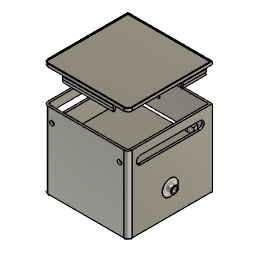
Chassis - Blank (Autodesk Fusion 360 design; units mm, degrees)
Autodesk Fusion 360 part; units mm, degrees
sketch "Floors" plane through (0, 0, 0) normal (0, 1, 0) x (1, 0, 0)
  line L0 (125, 0) -> (175, 0)
  line L1 (125, 2.5) -> (150, 2.5) construction
  line L2 (125, -23) -> (175, -23)
  line L3 (125, -20.5) -> (150, -20.5) construction
  line L4 (125, -22) -> (150, -22) construction
  line L5 (125, -35.125) -> (175, -35.125)
  line L6 (125, -36.725) -> (150, -36.725) construction
  line L7 (125, -36.125) -> (150, -36.125) construction
  line L8 (125, -55) -> (175, -55)
  line L9 (125, -52.5) -> (150, -52.5) construction
  line L10 (125, -62.5) -> (150, -62.5) construction
  line L11 (125, -90) -> (175, -90)
  line L12 (120, -130) -> (180, -130) construction
  line L13 (150, -4) -> (125, -4) construction
  line L14 (150, 1) -> (125, 1) construction
  line L15 (125, 3.5) -> (150, 3.5)
  dimension "d1" = 2.5
  dimension "d9" = 23
  dimension "d10" = 2.5
  dimension "d11" = 1
  dimension "d12" = 12.125
  dimension "d13" = 1
  dimension "d14" = 1.6
  dimension "d15" = 55
  dimension "d16" = 2.5
  dimension "d17" = 7.5
  dimension "d18" = 90
  dimension "d28" = 4
  dimension "d29" = 1
  dimension "d170" = 1
  constraint horizontal L0
  constraint horizontal L1
  constraint horizontal L2
  constraint parallel L2 L3
  constraint parallel L3 L4
  constraint horizontal L5
  constraint horizontal L6
  constraint horizontal L7
  constraint horizontal L8
  constraint horizontal L9
  constraint horizontal L10
  constraint horizontal L11
  constraint parallel L11 L12
  constraint parallel L5 L13
  constraint parallel L1 L14
  constraint horizontal L15
  measures "d1" distance of L0 L1
  measures "d9" distance of L0 L2
  measures "d10" distance of L2 L3
  measures "d11" distance of L2 L4
  measures "d12" distance of L2 L5
  measures "d13" distance of L5 L7
  measures "d14" distance of L5 L6
  measures "d15" distance of L0 L8
  measures "d16" distance of L8 L9
  measures "d17" distance of L8 L10
  measures "d18" distance of L0 L11
  measures "d28" distance of L0 L13
  measures "d29" distance of L0 L14
  measures "d170" distance of L1 L15
sketch "Base" plane through (0, 0, 0) normal (0, 0, 1) x (1, 0, 0)
  line L0 (-50, 50) -> (50, 50)
  line L1 (50, 50) -> (50, -50)
  line L2 (50, -50) -> (-50, -50)
  line L3 (-50, -50) -> (-50, 50)
  line L4 (-50, 50) -> (50, -50) construction
  line L5 (50, 50) -> (-50, -50) construction
  line L6 (47.5, -47.5) -> (-47.5, -47.5)
  line L7 (-47.5, -47.5) -> (-47.5, 47.5)
  line L8 (-47.5, 47.5) -> (47.5, 47.5)
  line L9 (47.5, 47.5) -> (47.5, -47.5)
  line L10 (47.5, -47.5) -> (-47.5, 47.5) construction
  line L11 (-47.5, -47.5) -> (47.5, 47.5) construction
  dimension "d4" = 100
  dimension "d6" = 95
  constraint horizontal L0
  constraint perpendicular L0 L1
  constraint parallel L0 L2
  constraint parallel L1 L3
  constraint coincident L4 origin
  constraint coincident L5 origin
  constraint horizontal L6
  constraint perpendicular L6 L7
  constraint parallel L6 L8
  constraint parallel L7 L9
  constraint coincident L10 origin
  constraint coincident L11 origin
  constraint coincident L4 L6.start
  constraint equal L0 L3
  measures "d4" distance of L0.start L0.end
  measures "d6" distance of L7.end L8.end
extrude "Extrude1" add sketch "Base" against normal up to surface (2.5 mm away) contours L0 L1 L2 L3 | L6 L7 L8 L9 makes body 1
extrude "Extrude2" add sketch "Base" along normal up to surface (90 mm away) bodies 1
fillet "Fillet1" radius 5 2 edges at (-50, -50, 43.75) (50, -50, 43.75) on bodies 1
sketch "Battery Mount" plane through (0, 0, 0) normal (0, 0, 1) x (1, 0, 0)
  line L0 (-15.5, 30) -> (15.5, 30)
  line L1 (15.5, 30) -> (15.5, -30)
  line L2 (15.5, -30) -> (-15.5, -30)
  line L3 (-15.5, -30) -> (-15.5, 30)
  line L4 (-15.5, 30) -> (15.5, -30) construction
  line L5 (15.5, 30) -> (-15.5, -30) construction
  line L6 (17.5, 32) -> (-17.5, 32)
  line L7 (-17.5, 32) -> (-17.5, -32)
  line L8 (-17.5, -32) -> (17.5, -32)
  line L9 (17.5, -32) -> (17.5, 32)
  line L10 (17.5, 32) -> (-17.5, -32) construction
  line L11 (-17.5, 32) -> (17.5, -32) construction
  line L12 (15.5, 30) -> (15.5, 32)
  line L13 (-15.5, 30) -> (-15.5, 32)
  dimension "d23" = 31
  dimension "d24" = 60
  dimension "d26" = 2
  dimension "d27" = 2
  constraint horizontal L0
  constraint perpendicular L0 L1
  constraint parallel L0 L2
  constraint parallel L1 L3
  constraint coincident L4 origin
  constraint coincident L5 origin
  constraint horizontal L6
  constraint perpendicular L6 L7
  constraint parallel L6 L8
  constraint parallel L7 L9
  constraint coincident L10 origin
  constraint coincident L11 origin
  constraint coincident L6 L12.end
  constraint perpendicular L6 L12
  constraint coincident L6 L13.end
  constraint perpendicular L6 L13
  measures "d23" distance of L1.end L2.end
  measures "d24" distance of L0.start L2.end
  measures "d26" distance of L1 L9
  measures "d27" distance of L0 L6
extrude "Extrude3" add sketch "Battery Mount" along normal up to surface (23 mm away) contours L1 L2 L3 L6 L7 L8 L9 L12 L13 bodies 1
extrude "Extrude4" add sketch "Battery Mount" along normal up to surface (4 mm away) contours L0 L6 L12 L13 bodies 1
extrude "Extrude5" cut sketch "Battery Mount" against normal up to surface (1 mm away) contours L0 L1 L2 L3 bodies 1
fillet "Fillet2" radius 1 2 edges at (-15.5, 0, -1) (15.5, 0, -1) on bodies 1
sketch "Motor Mount" plane through (0, 0, 23) normal (0, 0, 1) x (-1, 0, 0)
  line L0 (-17.5, -32) -> (-15.5, -32)
  line L1 (-15.5, -32) -> (-15.5, 30)
  line L2 (-15.5, 30) -> (15.5, 30)
  line L3 (15.5, 30) -> (15.5, -32)
  line L4 (15.5, -32) -> (17.5, -32)
  line L5 (17.5, -32) -> (17.5, 32)
  line L6 (17.5, 32) -> (-17.5, 32)
  line L7 (-17.5, 32) -> (-17.5, -32)
  line L8 (-17.5, 32) -> (-17.5, -32)
  line L9 (0, 0) -> (-65, 0)
  line L10 (-47.5, 0) -> (-47.5, 5.0625)
  line L11 (-47.5, 0) -> (-47.5, -5.0625)
  line L12 (-21, 5.0625) -> (-21, 0)
  line L13 (-47.5, 6.6625) -> (-17.5, 6.6625)
  line L14 (-47.5, 5.0625) -> (-21, 5.0625)
  line L15 (-45.5, 5.0625) -> (-45.5, 0)
  line L16 (-44.5, 5.8625) -> (-36.5, 5.8625)
  line L17 (-44.5, 5.8625) -> (-44.5, 0)
  line L18 (-36.5, 5.8625) -> (-36.5, 0)
  line L19 (-47.5, -47.9438) -> (-47.5, 49.8508) construction
  line L20 (-50, -50) -> (-50, 50)
  line L21 (-21, -5.0625) -> (-21, 0)
  line L22 (-47.5, -5.0625) -> (-21, -5.0625)
  line L23 (-47.5, -6.6625) -> (-17.5, -6.6625)
  line L24 (-17.5, -32) -> (-17.5, 32)
  line L25 (-36.5, -5.8625) -> (-36.5, 0)
  line L26 (-44.5, -5.8625) -> (-36.5, -5.8625)
  line L27 (-44.5, -5.8625) -> (-44.5, 0)
  line L28 (-45.5, -5.0625) -> (-45.5, 0)
  line L29 (-47.5, 0) -> (-47.5, -5.0625)
  line L30 (0, 0) -> (0, 50)
  line L31 (47.5, 6.6625) -> (17.5, 6.6625)
  line L32 (17.5, 32) -> (17.5, -32)
  line L33 (47.5, -6.6625) -> (17.5, -6.6625)
  line L34 (47.5, -5.0625) -> (21, -5.0625)
  line L35 (21, -5.0625) -> (21, 0)
  line L36 (21, 5.0625) -> (21, 0)
  line L37 (47.5, 5.0625) -> (21, 5.0625)
  line L38 (44.5, 5.8625) -> (36.5, 5.8625)
  line L39 (36.5, 5.8625) -> (36.5, 0)
  line L40 (36.5, -5.8625) -> (36.5, 0)
  line L41 (44.5, -5.8625) -> (36.5, -5.8625)
  line L42 (44.5, -5.8625) -> (44.5, 0)
  line L43 (45.5, -5.0625) -> (45.5, 0)
  line L44 (47.5, 0) -> (47.5, -5.0625)
  line L45 (47.5, 0) -> (47.5, 5.0625)
  line L46 (45.5, 5.0625) -> (45.5, 0)
  line L47 (44.5, 5.8625) -> (44.5, 0)
  line L48 (-47.5, 6.6625) -> (-47.5, 5.0625)
  line L49 (-47.5, -5.0625) -> (-47.5, -6.6625)
  line L50 (47.5, 6.6625) -> (47.5, 5.0625)
  line L51 (47.5, -5.0625) -> (47.5, -6.6625)
  line L52 (-21, 5.0625) -> (-21, 6.6625)
  line L53 (-21, -5.0625) -> (-21, -6.6625)
  line L54 (21, -5.0625) -> (21, -6.6625)
  line L55 (21, 5.0625) -> (21, 6.6625)
  dimension "d38" = 10.125
  dimension "d39" = 26.5
  dimension "d40" = 1.6
  dimension "d41" = 2
  dimension "d42" = 0.8
  dimension "d43" = 3
  dimension "d44" = 8
  dimension "d45" = 2.5
  constraint coincident L6.end L7.start
  constraint coincident L0.start L7.end
  constraint coincident L9.start L30.start
  constraint perpendicular L3 L9
  constraint coincident L9 L10.start
  constraint perpendicular L9 L10
  constraint perpendicular L9 L11
  constraint equal L10 L11
  constraint vertical L12
  constraint horizontal L13
  constraint coincident L8 L13.end
  constraint coincident L9 L12.end
  constraint coincident L9 L15.end
  constraint perpendicular L9 L15
  constraint parallel L13 L16
  constraint horizontal L14
  constraint perpendicular L14 L17
  constraint coincident L14 L15.start
  constraint coincident L9 L18.end
  constraint perpendicular L9 L18
  constraint coincident L10.start L19
  constraint symmetric L6.end L9 L0.start
  constraint symmetric L0.start L9 L6.end
  constraint symmetric L9 L10.start L11.start
  constraint symmetric L9 L10.end L11.end
  constraint symmetric L9 L12.start L21.start
  constraint symmetric L9 L12.end L21.end
  constraint symmetric L9 L13.start L23.start
  constraint symmetric L9 L13.end L23.end
  constraint symmetric L9 L15.start L28.start
  constraint symmetric L9 L15.end L28.end
  constraint symmetric L9 L16.start L26.start
  constraint symmetric L9 L16.end L25.start
  constraint symmetric L9 L17.end L27.end
  constraint symmetric L9 L18.end L25.end
  constraint perpendicular L6 L30
  constraint symmetric L6.end L30 L5.end
  constraint symmetric L0.start L30 L4.end
  constraint symmetric L10.start L30 L44.start
  constraint symmetric L10.end L30 L37.start
  constraint symmetric L11.end L30 L34.start
  constraint symmetric L12.start L30 L36.start
  constraint symmetric L12.end L30 L35.end
  constraint symmetric L13.start L30 L31.start
  constraint symmetric L13.end L30 L31.end
  constraint symmetric L15.start L30 L46.start
  constraint symmetric L15.end L30 L43.end
  constraint symmetric L16.start L30 L38.start
  constraint symmetric L16.end L30 L38.end
  constraint symmetric L17.end L30 L42.end
  constraint symmetric L18.end L30 L39.end
  constraint symmetric L21.start L30 L34.end
  constraint symmetric L23.start L30 L33.start
  constraint symmetric L23.end L30 L33.end
  constraint symmetric L25.start L30 L40.start
  constraint symmetric L26.start L30 L41.start
  constraint symmetric L28.start L30 L43.start
  constraint coincident L13 L52.end
  constraint perpendicular L13 L52
  constraint coincident L23 L53.end
  constraint perpendicular L23 L53
  constraint coincident L33 L54.end
  constraint perpendicular L33 L54
  constraint coincident L31 L55.end
  constraint perpendicular L31 L55
  measures "d38" distance of L10.end L11.end
  measures "d39" distance of L10 L12
  measures "d40" distance of L10.end L13
  measures "d41" distance of L10 L15
  measures "d42" distance of L14 L16
  measures "d43" distance of L10 L16.start
  measures "d44" distance of L17 L18
  measures "d45" distance of L19 L20
extrude "Extrude6" add sketch "Motor Mount" against normal up to surface (2.5 mm away) contours L7 L8 L9 L21 L23 L24 L53 | L7 L8 L9 L12 L13 L24 L52 | L22 L23 L25 L26 L27 L49 L53 | L9 L21 L22 L25 | L9 L12 L14 L18 | L13 L14 L16 L17 L18 L48 L52 | L9 L22 L25 L27 | L9 L14 L17 L18 | L9 L11 L22 L28 L29 | L22 L25 L26 L27 | L9 L22 L27 L28 | L9 L14 L15 L17 | L14 L16 L17 L18 | L9 L10 L14 L15 | L5 L31 L32 L33 L35 L36 L54 L55 | L31 L37 L38 L39 L47 L50 L55 | L33 L34 L40 L41 L42 L51 L54 | L34 L35 L36 L37 L39 L40 | L34 L37 L43 L44 L45 L46 | L37 L38 L39 L47 | L34 L37 L39 L40 L42 L47 | L34 L40 L41 L42 | L34 L37 L42 L43 L46 L47 bodies 1
extrude "Extrude7" add sketch "Motor Mount" along normal up to surface (13.725 mm away) contours L22 L23 L25 L26 L27 L49 L53 | L9 L21 L22 L25 | L9 L12 L14 L18 | L13 L14 L16 L17 L18 L48 L52 | L9 L22 L25 L27 | L9 L14 L17 L18 | L9 L11 L22 L28 L29 | L22 L25 L26 L27 | L9 L22 L27 L28 | L9 L14 L15 L17 | L14 L16 L17 L18 | L9 L10 L14 L15 | L31 L37 L38 L39 L47 L50 L55 | L33 L34 L40 L41 L42 L51 L54 | L34 L35 L36 L37 L39 L40 | L34 L37 L43 L44 L45 L46 | L37 L38 L39 L47 | L34 L37 L39 L40 L42 L47 | L34 L40 L41 L42 | L34 L37 L42 L43 L46 L47 bodies 1
extrude "Extrude8" cut sketch "Motor Mount" along normal up to surface (12.125 mm away) contours L9 L21 L22 L25 | L9 L12 L14 L18 | L9 L22 L25 L27 | L9 L14 L17 L18 | L22 L25 L26 L27 | L9 L22 L27 L28 | L9 L14 L15 L17 | L14 L16 L17 L18 | L34 L35 L36 L37 L39 L40 | L37 L38 L39 L47 | L34 L37 L39 L40 L42 L47 | L34 L40 L41 L42 | L34 L37 L42 L43 L46 L47 bodies 1
extrude "Extrude9" cut sketch "Motor Mount" along normal up to surface (13.125 mm away) and the other way up to surface (1 mm away) contours L9 L22 L25 L27 | L9 L14 L17 L18 | L22 L25 L26 L27 | L14 L16 L17 L18 | L37 L38 L39 L47 | L34 L37 L39 L40 L42 L47 | L34 L40 L41 L42 bodies 1
sketch "Motor Hole" plane through (0, 0, 0) normal (1, 0, 0) x (0, 1, 0)
  line L0 (-5.0625, 35.125) -> (5.0625, 35.125)
  line L1 (5.0625, 35.125) -> (5.0625, 23)
  line L2 (-5.0625, 23) -> (-5.0625, 35.125)
  line L3 (-5.0625, 23) -> (0, 23)
  line L4 (5.0625, 23) -> (0, 23)
  line L5 (0, 35.125) -> (0, 23)
  line L6 (5.0625, 29.0625) -> (-5.0625, 29.0625)
  circle A0 centre (0, 29.0625) radius 2.25
  dimension "d56" = 4.5
  constraint midpoint L0 L5.start
  constraint coincident L3.end L4.end
  constraint midpoint L1 L6.start
  constraint midpoint L2 L6.end
  constraint midpoint L6 A0.centre
  measures "d56" diameter of A0
extrude "Extrude10" cut sketch "Motor Hole" along normal through all and the other way through all contours L5 L6 A0 | L5 L6 A0 | L5 L6 A0 | L5 L6 A0 bodies 1
sketch "Hub Support - L" plane through (50, 0, 0) normal (1, 0, 0) x (0, 1, 0)
  circle A0 centre (0, 29.0625) radius 2.25
  line L0 (-45, 90) -> (-45, -2.5)
  line L1 (-45, -2.5) -> (50, -2.5)
  line L2 (50, -2.5) -> (50, 90)
  line L3 (50, 90) -> (-45, 90)
  circle A1 centre (0, 29.0625) radius 4.5
  circle A2 centre (0, 29.0625) radius 3.25
  point P0 (0, 29.0625)
  dimension "d59" = 9
  dimension "d60" = 6.5
  constraint coincident P0 A0.centre
  measures "d59" diameter of A1
  measures "d60" diameter of A2
extrude "Extrude11" add sketch "Hub Support - L" along normal blind 5 contours A1 bodies 1
sketch "Hub Support - R" plane through (-50, 0, 0) normal (-1, 0, 0) x (0, -1, 0)
  circle A0 centre (0, 29.0625) radius 2.25
  line L0 (45, -2.5) -> (45, 90)
  line L1 (45, 90) -> (-50, 90)
  line L2 (-50, 90) -> (-50, -2.5)
  line L3 (-50, -2.5) -> (45, -2.5)
  circle A1 centre (0, 29.0625) radius 4.5
  circle A2 centre (0, 29.0625) radius 3.25
  dimension "d63" = 6.5
  dimension "d64" = 9
  constraint concentric A0 A1
  constraint concentric A1 A2
  measures "d63" diameter of A2
  measures "d64" diameter of A1
extrude "Extrude12" add sketch "Hub Support - R" along normal blind 5 contours A1 bodies 1
extrude "Extrude13" cut sketch "Hub Support - R" against normal blind 2.5 contours A0 | A2 bodies 1
fillet "Fillet3" radius 5 2 edges at (-50, 4.1955, 30.6898) (50, -4.1955, 30.6898) on bodies 1
sketch "Cable Holders" plane through (0, 0, 36.725) normal (0, 0, 1) x (-1, 0, 0)
  line L0 (-47.5, -6.6625) -> (-21, -6.6625)
  line L1 (-21, -6.6625) -> (-21, 6.6625)
  line L2 (-21, 6.6625) -> (-47.5, 6.6625)
  line L3 (-47.5, 6.6625) -> (-47.5, -6.6625)
  line L4 (-47.5, 6.6625) -> (-21, 6.6625)
  line L5 (-47.5, -6.6625) -> (-47.5, 6.6625)
  line L6 (-21, -6.6625) -> (-47.5, -6.6625)
  line L7 (21, 6.6625) -> (47.5, 6.6625)
  line L8 (47.5, -6.6625) -> (21, -6.6625)
  line L9 (47.5, 6.6625) -> (47.5, -6.6625)
  line L10 (-46.375, 6.6625) -> (-46.375, -6.6625)
  line L11 (46.375, 6.6625) -> (46.375, -6.6625)
  line L12 (-40, 6.6625) -> (-40, -6.6625)
  line L13 (40, 6.6625) -> (40, -6.6625)
  line L14 (37, 6.6625) -> (37, -6.6625)
  line L15 (-37, 6.6625) -> (-37, -6.6625)
  dimension "d71" = 1.125
  dimension "d72" = 1.125
  dimension "d73" = 7.5
  dimension "d74" = 7.5
  dimension "d75" = 3
  dimension "d76" = 3
  constraint coincident L4 L10.start
  constraint coincident L6 L10.end
  constraint perpendicular L6 L10
  constraint coincident L7 L11.start
  constraint coincident L8 L11.end
  constraint perpendicular L8 L11
  constraint coincident L4 L12.start
  constraint coincident L6 L12.end
  constraint perpendicular L6 L12
  constraint coincident L7 L13.start
  constraint coincident L8 L13.end
  constraint perpendicular L8 L13
  constraint coincident L7 L14.start
  constraint coincident L8 L14.end
  constraint perpendicular L8 L14
  constraint coincident L4 L15.start
  constraint coincident L6 L15.end
  constraint perpendicular L6 L15
  measures "d71" distance of L3 L10
  measures "d72" distance of L9 L11
  measures "d73" distance of L5 L12
  measures "d74" distance of L9 L13
  measures "d75" distance of L12 L15
  measures "d76" distance of L13 L14
extrude "Extrude14" add sketch "Cable Holders" along normal blind 10 contours L0 L2 L4 L6 L10 L12 | L0 L2 L4 L6 L12 L15 | L7 L8 L13 L14 | L7 L8 L11 L13 bodies 1
extrude "Extrude15" cut sketch "Cable Holders" along normal blind 7 contours L0 L2 L4 L6 L10 L12 | L7 L8 L11 L13 bodies 1
chamfer "Chamfer1" distance 1 distance2 7.5 1 edges at (37, 0, 36.725) measured on face at (31.6667, -2.2208, 36.725) on bodies 1
chamfer "Chamfer2" distance 1 distance2 7.5 1 edges at (-37, 0, 36.725) measured on face at (-26.3333, 2.2208, 36.725) on bodies 1
sketch "Access Hole" plane through (0, 47.5, 0) normal (0, 1, 0) x (-1, 0, 0)
  line L0 (-47.5, 0) -> (47.5, 0)
  line L1 (-47.5, 0) -> (-47.5, 90)
  line L2 (47.5, 0) -> (47.5, 90)
  line L3 (-125, 52.5) -> (-150, 52.5)
  line L4 (-42.5, 90) -> (-42.5, 0)
  line L5 (42.5, 90) -> (42.5, 0)
  line L6 (-125, 52.5) -> (47.5, 52.5)
  line L7 (-47.5, 90) -> (47.5, 90)
  line L8 (47.5, 90) -> (47.5, 0)
  line L9 (47.5, 0) -> (-47.5, 0)
  line L10 (-47.5, 0) -> (-47.5, 90)
  dimension "d85" = 5
  dimension "d86" = 5
  constraint coincident L0 L4.end
  constraint perpendicular L0 L4
  constraint coincident L0 L5.end
  constraint perpendicular L0 L5
  constraint coincident L3.start L6.start
  constraint coincident L2 L6.end
  constraint perpendicular L2 L6
  measures "d85" distance of L1 L4
  measures "d86" distance of L2 L5
extrude "Extrude16" cut sketch "Access Hole" along normal blind 20 contours L0 L4 L5 L6 L9 bodies 1
fillet "Fillet4" radius 10 4 edges at (42.5, 48.75, 0) (-42.5, 48.75, 0) (42.5, 48.75, 52.5) (-42.5, 48.75, 52.5) on bodies 1
sketch "Zip Tie Holes" plane through (0, 0, 0) normal (0, 0, 1) x (-1, 0, 0)
  line L0 (17.5, -32) -> (-17.5, -32)
  line L1 (-17.5, -32) -> (-17.5, 32)
  line L2 (-17.5, 32) -> (17.5, 32)
  line L3 (17.5, 32) -> (17.5, -32)
  line L4 (32.5, -50) -> (32.5, -47.5)
  line L5 (32.5, -47.5) -> (47.5, -47.5)
  line L6 (47.5, -47.5) -> (47.5, 47.5)
  line L7 (47.5, 47.5) -> (-47.5, 47.5)
  line L8 (-47.5, 47.5) -> (-47.5, -47.5)
  line L9 (-47.5, -47.5) -> (-32.5, -47.5)
  line L10 (-32.5, -47.5) -> (-32.5, -50)
  line L11 (-32.5, -50) -> (32.5, -50)
  line L12 (-47.5, 47.5) -> (-47.5, -47.5)
  line L13 (-47.5, -47.5) -> (-32.5, -47.5)
  line L14 (-42.5, -36.5) -> (-37.5, -36.5)
  line L15 (-37.5, -36.5) -> (-37.5, -41.5)
  line L16 (-37.5, -41.5) -> (-42.5, -41.5)
  line L17 (-42.5, -41.5) -> (-42.5, -36.5)
  line L18 (-27.5, -36.5) -> (-22.5, -36.5)
  line L19 (-22.5, -36.5) -> (-22.5, -41.5)
  line L20 (-22.5, -41.5) -> (-27.5, -41.5)
  line L21 (-27.5, -41.5) -> (-27.5, -36.5)
  dimension "d91" = 11
  dimension "d92" = 5
  dimension "d93" = 5
  dimension "d94" = 20
  constraint horizontal L14
  constraint vertical L15
  constraint horizontal L16
  constraint vertical L17
  constraint horizontal L18
  constraint vertical L19
  constraint horizontal L20
  constraint vertical L21
  constraint collinear L14 L18
  constraint collinear L16 L20
  constraint equal L14 L17
  constraint equal L14 L18
  measures "d91" distance of L13 L14
  measures "d92" distance of L12 L17
  measures "d93" distance of L18 L20
  measures "d94" distance of L17 L19
extrude "Extrude17" cut sketch "Zip Tie Holes" against normal through all contours L14 L15 L16 L17 | L18 L19 L20 L21 bodies 1
sketch "Switch Mount" plane through (0, 41.5, 0) normal (0, -1, 0) x (1, 0, 0)
  line L0 (22.5, -2.5) -> (27.5, -2.5)
  line L1 (27.5, -2.5) -> (27.5, 0)
  line L2 (27.5, 0) -> (22.5, 0)
  line L3 (22.5, 0) -> (22.5, -2.5)
  line L4 (37.5, 0) -> (42.5, 0)
  line L5 (22.5, 0) -> (27.5, 0)
  line L6 (37.5, 0) -> (37.5, 2)
  line L7 (37.5, 2) -> (27.5, 2)
  line L8 (27.5, 2) -> (27.5, 0)
  circle A0 centre (32.5, 12) radius 10
  line L9 (27.5, 2) -> (27.5, 3.3397)
  line L10 (37.5, 2) -> (37.5, 3.3397)
  line L11 (37.5, 0) -> (27.5, 0)
  point P0 (32.5, 2)
  point P1 (32.5, 2)
  dimension "d96" = 2
  dimension "d97" = 20
  constraint coincident L4.start L6.start
  constraint perpendicular L4 L6
  constraint perpendicular L6 L7
  constraint perpendicular L5 L8
  constraint coincident L1.end L2.start
  constraint midpoint L7 P1
  constraint coincident A0 P1
  constraint vertical A0.centre P1
  constraint coincident P1 P0
  constraint coincident A0 L9.end
  constraint perpendicular L7 L9
  constraint coincident A0 L10.end
  constraint perpendicular L7 L10
  measures "d96" distance of L4.start L6.end
  measures "d97" diameter of A0
extrude "Extrude18" add sketch "Switch Mount" along normal blind 10 contours L6 L7 L8 L11 | L7 A0 L9 | L7 A0 L10 bodies 1
fillet "Fillet5" radius 0.5 6 edges at (37.5, 36.5, 3.3397) (27.5, 36.5, 3.3397) (27.5, 34, 0) (37.5, 34, 0) (32.5, 31.5, 0) (32.5, 31.5, 2) on bodies 1
ref_plane "WorkPlane1" through (0, 1.25, 55) normal (0, 0, 1) x (1, 0, 0)
sketch "Bread Board Mount" plane through (0, 0, 55) normal (0, 0, 1) x (1, 0, 0)
  line L0 (-47.5, -47.5) -> (47.5, -47.5)
  line L1 (47.5, -47.5) -> (47.5, 47.5)
  line L2 (-47.5, 47.5) -> (-47.5, -47.5)
  line L3 (47.5, 47.5) -> (-47.5, 47.5)
  line L4 (0, -47.5) -> (0, 47.5)
  line L5 (-47.5, 0) -> (47.5, 0)
  line L6 (-41, 41.5) -> (41, 41.5)
  line L7 (41, 41.5) -> (41, -41.5)
  line L8 (41, -41.5) -> (-41, -41.5)
  line L9 (-41, -41.5) -> (-41, 41.5)
  line L10 (-41, 41.5) -> (41, -41.5) construction
  line L11 (41, 41.5) -> (-41, -41.5) construction
  circle A0 centre (47.5, -47.5) radius 20
  circle A1 centre (-47.5, -47.5) radius 20
  circle A2 centre (47.5, 47.5) radius 20
  circle A3 centre (-47.5, 47.5) radius 20
  circle A4 centre (47.5, -47.5) radius 12.5
  circle A5 centre (-47.5, -47.5) radius 12.5
  circle A6 centre (47.5, 47.5) radius 12.5
  circle A7 centre (-47.5, 47.5) radius 12.5
  dimension "d104" = 83
  dimension "d105" = 82
  dimension "d106" = 40
  dimension "d107" = 25
  constraint midpoint L0 L4.start
  constraint midpoint L3 L4.end
  constraint midpoint L2 L5.start
  constraint midpoint L1 L5.end
  constraint horizontal L6
  constraint perpendicular L6 L7
  constraint parallel L6 L8
  constraint parallel L7 L9
  constraint coincident L10 origin
  constraint coincident L11 origin
  constraint coincident L0.end L1.start
  constraint coincident L0.start L2.end
  constraint coincident L1.end L3.start
  constraint coincident L2.start L3.end
  constraint equal A2 A3
  constraint equal A0 A2
  constraint equal A0 A1
  constraint concentric A0 A4
  constraint concentric A2 A6
  constraint concentric A3 A7
  constraint equal A6 A7
  constraint equal A4 A6
  constraint equal A4 A5
  measures "d104" distance of L6 L8
  measures "d105" distance of L7 L9
  measures "d106" diameter of A1
  measures "d107" diameter of A5
extrude "Extrude19" add sketch "Bread Board Mount" against normal up to surface (2.5 mm away) contours L0 L8 A1 A5 | L2 L9 A1 A5 | L8 L9 A1 A5 | L4 L5 L8 L9 A1 | L0 L8 A0 A4 | L4 L5 L7 L8 A0 | L2 L9 A3 A7 | L4 L5 L6 L9 A3 | L7 L8 A0 A4 | L4 L5 L6 L7 A2 | L3 L6 A3 A7 | L6 L9 A3 A7 | L1 L7 A0 A4 | L3 L6 A2 A6 | L6 L7 A2 A6 | L1 L7 A2 A6 bodies 1
extrude "Extrude20" add sketch "Bread Board Mount" along normal up to surface (7.5 mm away) contours L0 L8 A1 A5 | L2 L9 A1 A5 | L0 L8 A0 A4 | L2 L9 A3 A7 | L3 L6 A3 A7 | L1 L7 A0 A4 | L3 L6 A2 A6 | L1 L7 A2 A6 bodies 1
fillet "Fillet6" radius 2.5 32 edges at (50, 2.5, -2.5) (48.5355, -48.5355, -2.5) (0, -50, -2.5) (-48.5355, -48.5355, -2.5) (-50, 2.5, -2.5) (-47.5, -47.5, 45) (47.5, -47.5, 45) (47.5, 0, 0) (0, -47.5, 0) (-47.5, 0, 0) (-47.5, 0, 20.5) (-17.5, 0, 20.5) (47.5, 0, 20.5) (17.5, 0, 20.5) (-37, 0, 46.725) (-36, 0, 36.725) (-46.375, 0, 46.725) (-40, 0, 43.725) (-40, 0, 36.725) (36, 0, 36.725) (40, 0, 36.725) (37, 0, 46.725) (46.375, 0, 46.725) (40, 0, 43.725) (17.5, 0, 0) (-17.5, 0, 0) (47.5, -31.25, 52.5) (31.25, -47.5, 52.5) (-31.25, -47.5, 52.5) (-47.5, -31.25, 52.5) (47.5, 31.25, 52.5) (-47.5, 31.25, 52.5) on bodies 1
sketch "Skid Pads" plane through (0, 0, -2.5) normal (0, 0, -1) x (1, 0, 0)
  line L0 (-47.5, 45) -> (-47.5, -50)
  line L1 (-47.5, -50) -> (47.5, -50)
  line L2 (47.5, -50) -> (47.5, 45)
  arc A0 (47.5, 45) -> (45, 47.5) centre (45, 45) ccw
  line L3 (45, 47.5) -> (-45, 47.5)
  arc A1 (-45, 47.5) -> (-47.5, 45) centre (-45, 45) ccw
  line L4 (42.5, -36.5) -> (42.5, -41.5)
  line L5 (42.5, -41.5) -> (37.5, -41.5)
  line L6 (37.5, -41.5) -> (37.5, -36.5)
  line L7 (37.5, -36.5) -> (42.5, -36.5)
  line L8 (27.5, -36.5) -> (27.5, -41.5)
  line L9 (27.5, -41.5) -> (22.5, -41.5)
  line L10 (22.5, -41.5) -> (22.5, -36.5)
  line L11 (22.5, -36.5) -> (27.5, -36.5)
  line L12 (47.5, 45) -> (47.5, -47.5)
  line L13 (-45, 47.5) -> (45, 47.5)
  line L14 (-47.5, -47.5) -> (-47.5, 45)
  line L15 (47.5, -47.5) -> (-47.5, -47.5)
  line L16 (0, 47.5) -> (0, -47.5)
  circle A2 centre (0, -43.5) radius 4
  circle A3 centre (0, 43.5) radius 4
  point P0 (0, -47.5)
  point P1 (0, 47.5)
  dimension "d114" = 8
  constraint midpoint L13 P1
  constraint midpoint L15 P0
  constraint coincident L16 A2.centre
  constraint coincident L16 A3.centre
  constraint equal A2 A3
  constraint coincident A2 P0
  constraint coincident L16 P0
  constraint coincident P0 L16.end
  constraint coincident A3 P1
  constraint coincident L16 P1
  constraint coincident P1 L16.start
  measures "d114" diameter of A2
extrude "Extrude21" add sketch "Skid Pads" along normal up to surface (1 mm away) contours L16 A2 | L16 A2 | L16 A3 | L16 A3 bodies 1
fillet "Fillet7" radius 4 2 edges at (-3.7293, 42.0535, -3.5) (-3.7293, -44.9465, -3.5) on bodies 1
fillet "Fillet8" radius 1 2 edges at (-3.7293, 42.0535, -2.5) (-3.7293, -44.9465, -2.5) on bodies 1
sketch "Sight" plane through (50, 0, 0) normal (1, 0, 0) x (0, 1, 0)
  line L0 (-45, 0) -> (45, 0)
  line L1 (45, 0) -> (45, 90)
  line L2 (45, 90) -> (-45, 90)
  line L3 (-45, 90) -> (-45, 0)
  line L4 (50, 0) -> (50, 90)
  line L5 (-50, 90) -> (-50, 0)
  line L6 (-45, 90) -> (45, 90)
  line L7 (-40, 90) -> (-40, 22.1141)
  line L8 (40, 90) -> (40, 27.2483)
  line L9 (-43.441, 80) -> (42.5637, 80)
  line L10 (-42.9722, 70) -> (42.2086, 70)
  circle A0 centre (0, 29.0625) radius 9.5
  line L11 (-45, 0) -> (50, 0)
  line L12 (50, 0) -> (50, 90)
  line L13 (50, 90) -> (-45, 90)
  line L14 (-45, 90) -> (-45, 0)
  point P0 (-50, 90)
  point P1 (50, 90)
  dimension "d121" = 10
  dimension "d122" = 10
  dimension "d123" = 10
  dimension "d124" = 10
  constraint coincident L6 L7.start
  constraint perpendicular L6 L7
  constraint coincident L6 L8.start
  constraint perpendicular L6 L8
  constraint perpendicular L8 L9
  constraint perpendicular L8 L10
  measures "d121" distance of L5 L7
  measures "d122" distance of L4 L8
  measures "d123" distance of L2 L9
  measures "d124" distance of L9 L10
extrude "Extrude22" cut sketch "Sight" against normal through all and the other way blind 0 contours L7 L8 L9 L10 bodies 1
fillet "Fillet9" radius 5 16 edges at (-48.75, 40, 70) (48.75, 40, 70) (-48.75, 40, 70) (48.75, 40, 70) (-48.75, -40, 70) (48.75, -40, 70) (-48.75, -40, 70) (48.75, -40, 70) (48.75, -40, 80) (-48.75, -40, 80) (-48.75, 40, 80) (48.75, 40, 80) (-48.75, 40, 80) (48.75, 40, 80) (48.75, -40, 80) (-48.75, -40, 80) on bodies 1
sketch "LED Holes" plane through (0, 50, 0) normal (0, 1, 0) x (-1, 0, 0)
  line L0 (-32.5, 52.5) -> (32.5, 52.5)
  arc A0 (42.5, 42.5) -> (32.5, 52.5) centre (32.5, 42.5) ccw
  line L1 (42.5, 42.5) -> (42.5, 10)
  arc A1 (32.5, 0) -> (42.5, 10) centre (32.5, 10) ccw
  line L2 (32.5, 0) -> (-32.5, 0)
  arc A2 (-42.5, 10) -> (-32.5, 0) centre (-32.5, 10) ccw
  line L3 (-42.5, 10) -> (-42.5, 42.5)
  arc A3 (-32.5, 52.5) -> (-42.5, 42.5) centre (-32.5, 42.5) ccw
  arc A4 (47.5, -2.5) -> (50, 0) centre (47.5, 0) ccw
  line L4 (50, 0) -> (50, 90)
  line L5 (50, 90) -> (-50, 90)
  line L6 (-50, 90) -> (-50, 0)
  arc A5 (-50, 0) -> (-47.5, -2.5) centre (-47.5, 0) ccw
  line L7 (-47.5, -2.5) -> (47.5, -2.5)
  line L8 (50, 90) -> (-50, 90)
  line L9 (50, 80) -> (50, 70) construction
  line L10 (-50, 80) -> (-50, 70) construction
  line L11 (-50, 75) -> (50, 75) construction
  circle A6 centre (-40, 75) radius 2.6
  circle A7 centre (40, 75) radius 2.6
  point P0 (50, 70)
  point P1 (50, 80)
  point P2 (-50, 70)
  point P3 (-50, 80)
  dimension "d130" = 10
  dimension "d131" = 10
  dimension "d132" = 5.2
  constraint coincident P1 L9.start
  constraint coincident P0 L9.end
  constraint coincident P3 L10.start
  constraint coincident P2 L10.end
  constraint midpoint L10 L11.start
  constraint midpoint L9 L11.end
  constraint coincident L11 A6.centre
  constraint coincident L11 A7.centre
  constraint equal A6 A7
  measures "d130" distance of L10 A6.centre
  measures "d131" distance of L9 A7.centre
  measures "d132" diameter of A6
extrude "Extrude23" cut sketch "LED Holes" along normal blind 0 and the other way blind 100 contours A6 | A7 bodies 1
sketch "Programming Hole" plane through (0, 50, 0) normal (0, 1, 0) x (-1, 0, 0)
  circle A0 centre (-40, 75) radius 2.6
  circle A1 centre (40, 75) radius 2.6
  line L0 (-32.5, 52.5) -> (32.5, 52.5)
  arc A2 (42.5, 42.5) -> (32.5, 52.5) centre (32.5, 42.5) ccw
  line L1 (42.5, 42.5) -> (42.5, 10)
  arc A3 (32.5, 0) -> (42.5, 10) centre (32.5, 10) ccw
  line L2 (32.5, 0) -> (-32.5, 0)
  arc A4 (-42.5, 10) -> (-32.5, 0) centre (-32.5, 10) ccw
  line L3 (-42.5, 10) -> (-42.5, 42.5)
  arc A5 (-32.5, 52.5) -> (-42.5, 42.5) centre (-32.5, 42.5) ccw
  arc A6 (47.5, -2.5) -> (50, 0) centre (47.5, 0) ccw
  line L4 (50, 0) -> (50, 90)
  line L5 (50, 90) -> (-50, 90)
  line L6 (-50, 90) -> (-50, 0)
  arc A7 (-50, 0) -> (-47.5, -2.5) centre (-47.5, 0) ccw
  line L7 (-47.5, -2.5) -> (47.5, -2.5)
  line L8 (47.5, 2.5) -> (47.5, 90)
  line L9 (-47.5, 90) -> (47.5, 90)
  line L10 (36, 75) -> (10, 75)
  line L11 (10, 75) -> (10, 66)
  line L12 (10, 66) -> (36, 66)
  line L13 (36, 66) -> (36, 75)
  dimension "d137" = 26
  dimension "d138" = 11.5
  dimension "d139" = 9
  dimension "d140" = 15
  constraint horizontal L10
  constraint vertical L11
  constraint horizontal L12
  constraint vertical L13
  measures "d137" distance of L11.end L12.end
  measures "d138" distance of L8 L13
  measures "d139" distance of L10.end L11.end
  measures "d140" distance of L9 L10
extrude "Extrude24" cut sketch "Programming Hole" against normal blind 10 contours L10 L11 L12 L13 bodies 1
fillet "Fillet10" radius 1 4 edges at (-10, 48.75, 66) (-10, 48.75, 75) (-36, 48.75, 66) (-36, 48.75, 75) on bodies 1
ref_plane "WorkPlane2" through (0, 0, 130) normal (0, 0, 1) x (1, 0, 0)
sketch "Roof" plane through (0, 0, 130) normal (0, 0, 1) x (1, 0, 0)
  line L0 (45, -50) -> (-45, -50)
  arc A0 (-50, -45) -> (-45, -50) centre (-45, -45) ccw
  arc A1 (45, -50) -> (50, -45) centre (45, -45) ccw
  line L1 (50, 50) -> (50, -45)
  line L2 (-50, 50) -> (50, 50)
  line L3 (-50, -45) -> (-50, 50)
  line L4 (-47.5, 47.5) -> (-47.5, -45)
  line L5 (-45, -47.5) -> (45, -47.5)
  line L6 (47.5, 47.5) -> (-47.5, 47.5)
  line L7 (47.5, -45) -> (47.5, 47.5)
  arc A2 (45, -47.5) -> (47.5, -45) centre (45, -45) ccw
  arc A3 (-47.5, -45) -> (-45, -47.5) centre (-45, -45) ccw
  line L8 (30, -45) -> (-30, -45)
  line L9 (-30, -45) -> (-30, -47.5)
  line L10 (30, -45) -> (30, -47.5)
  line L11 (47.5, 17.8502) -> (45, 17.8502)
  line L12 (45, 17.8502) -> (45, 45)
  line L13 (45, 45) -> (15, 45)
  line L14 (15, 45) -> (15, 47.5)
  line L15 (-47.5, 17.8502) -> (-45, 17.8502)
  line L16 (-45, 17.8502) -> (-45, 45)
  line L17 (-45, 45) -> (-15, 45)
  line L18 (-15, 45) -> (-15, 47.5)
  point P0 (0, -47.5)
  point P1 (0, -45)
  dimension "d147" = 60
  dimension "d148" = 30
  dimension "d149" = 2.5
  constraint horizontal L8
  constraint coincident L5 L9.end
  constraint perpendicular L5 L9
  constraint coincident L5 L10.end
  constraint perpendicular L5 L10
  constraint coincident L7 L11.start
  constraint perpendicular L7 L11
  constraint perpendicular L11 L12
  constraint perpendicular L7 L13
  constraint coincident L6 L14.end
  constraint perpendicular L6 L14
  constraint coincident L4 L15.start
  constraint perpendicular L4 L15
  constraint perpendicular L15 L16
  constraint perpendicular L16 L17
  constraint coincident L6 L18.end
  constraint perpendicular L6 L18
  constraint collinear L13 L17
  constraint collinear L11 L15
  constraint midpoint L5 P0
  constraint midpoint L8 P1
  constraint vertical P0 P1
  constraint equal L13 L17
  constraint equal L11 L15
  constraint equal L9 L15
  constraint equal L11 L14
  measures "d147" distance of L8.start L8.end
  measures "d148" distance of L14 L18
  measures "d149" distance of L11.start L11.end
extrude "Extrude25" add sketch "Roof" along normal blind 2.5 separate body contours L0 A0 A1 L1 L2 L3 | L4 L6 L15 L16 L17 L18 | L4 L5 L6 L7 A2 A3 L8 L9 L10 L11 L12 L13 L14 L15 L16 L17 L18 | L6 L7 L11 L12 L13 L14 | L5 L8 L9 L10 makes body 2
extrude "Extrude26" add sketch "Roof" against normal blind 10 contours L4 L6 L15 L16 L17 L18 | L6 L7 L11 L12 L13 L14 | L5 L8 L9 L10 bodies 2
fillet "Fillet11" radius 2.5 7 edges at (0, -45, 130) (45, 31.4251, 130) (30, 45, 130) (-30, 45, 130) (-45, 31.4251, 130) (-47.5, 47.5, 125) (47.5, 47.5, 125) on bodies 2
fillet "Fillet12" radius 2.5 4 edges at (-44.2678, 44.2678, 129.2678) (-45, 45, 123.75) (44.2678, 44.2678, 129.2678) (45, 45, 123.75) on bodies 2
sketch "Roof Brim" plane through (0, 0, 132.5) normal (0, 0, 1) x (-1, 0, 0)
  arc A0 (-45, 50) -> (-50, 45) centre (-45, 45) ccw
  line L0 (-50, 45) -> (-50, -50)
  line L1 (-50, -50) -> (50, -50)
  line L2 (50, -50) -> (50, 45)
  arc A1 (50, 45) -> (45, 50) centre (45, 45) ccw
  line L3 (45, 50) -> (-45, 50)
  line L4 (45, 50) -> (-45, 50)
  arc A2 (-45, 50) -> (-50, 45) centre (-45, 45) ccw
  line L5 (-50, 45) -> (-50, -50)
  arc A3 (50, 45) -> (45, 50) centre (45, 45) ccw
  line L6 (50, -50) -> (50, 45)
  line L7 (-50, -50) -> (50, -50)
  line L8 (-49, 45) -> (-49, -49)
  line L9 (-49, -49) -> (49, -49)
  line L10 (49, -49) -> (49, 45)
  line L11 (-45, 49) -> (45, 49)
  arc A4 (-45, 49) -> (-49, 45) centre (-45, 45) ccw
  arc A5 (49, 45) -> (45, 49) centre (45, 45) ccw
  dimension "d158" = 1
  dimension "d159" = 1
  dimension "d160" = 1
  dimension "d161" = 1
  constraint parallel L5 L8
  constraint perpendicular L8 L9
  constraint perpendicular L9 L10
  constraint perpendicular L10 L11
  constraint tangent L11 A4
  constraint tangent L8 A4
  constraint tangent L11 A5
  constraint tangent L10 A5
  constraint coincident A0.centre A2.centre
  constraint coincident A1.centre A3.centre
  measures "d158" distance of L0 L8
  measures "d159" distance of L6 L10
  measures "d160" distance of L7 L9
  measures "d161" distance of L3 L11
extrude "Extrude27" add sketch "Roof Brim" along normal blind 1 bodies 2
chamfer "Chamfer3" distance 0.5 distance2 5 7 edges at (-30, 47.5, 120) (-47.5, 31.4251, 120) (-46.7678, 46.7678, 120) (30, 47.5, 120) (46.7678, 46.7678, 120) (47.5, 31.4251, 120) (0, -47.5, 120) measured on face at (-34.1667, 46.6667, 120) measured on face at (-34.1667, 46.6667, 120) measured on face at (-45.5894, 47.4295, 126.6667) measured on face at (34.1667, 46.6667, 120) measured on face at (45.5894, 47.4295, 126.6667) measured on face at (34.1667, 46.6667, 120) measured on face at (-10, -45.8333, 120) on bodies 2
fillet "Fillet13" radius 33 7 edges at (-47.5, 31.4251, 125) (-46.7678, 46.7678, 125) (-30, 47.5, 125) (30, 47.5, 125) (46.7678, 46.7678, 125) (47.5, 31.4251, 125) (0, -47.5, 125) on bodies 2
named bodies: "Chassis", "Roof"
